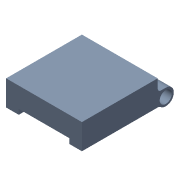
# Autodesk Inventor part: Rocker Box Top
Saved by Autodesk Inventor 2014 (Build 180170000, 170)
## iProperties
Created: 2013-05-18
Part Number: Rocker Box Top
Material: Generic
Document SubType Name: Modeling
Designer: richard
Density: 1 g/cm^3
Appearance: Light Steel Blue
Author: richard
Autodesk Inventor part; units mm, degrees
ref_plane "YZ Plane" through (0, 0, 0) normal (1, 0, 0) x (0, 1, 0)
ref_plane "XZ Plane" through (0, 0, 0) normal (0, 1, 0) x (-1, 0, 0)
ref_plane "XY Plane" through (0, 0, 0) normal (0, 0, 1) x (1, 0, 0)
sketch "Sketch1" plane through (0, 0, 0) normal (0, 0, 1) x (1, 0, 0)
  line L0 (-37.5, -5) -> (-25, -5)
  line L1 (-25, -5) -> (-25, 0)
  line L2 (-25, 0) -> (25, 0)
  line L3 (25, 0) -> (25, -5)
  line L4 (25, -5) -> (37.5, -5)
  line L5 (37.5, -5) -> (37.5, 20)
  line L6 (37.5, 20) -> (-37.5, 20)
  line L7 (-37.5, 20) -> (-37.5, -5)
  line L8 (0, 20) -> (0, 0) construction
  dimension "d0" = 50
  dimension "d1" = 75
  dimension "d2" = 25
  dimension "d3" = 5
  constraints: 18 end point, 5 parallel, 3 midpoint, 2 collinear, 2 perpendicular, 1 coincident, 1 horizontal, 1 other
  measures "d0" distance of L1.end L2.end
  measures "d1" distance between parallel lines of L5 L7
  measures "d2" distance between parallel lines of L6 L4
  measures "d3" distance of L2.end L3.end
extrude "Extrusion1" add sketch "Sketch1" along normal blind 75
sketch "Sketch2" plane through (-25, 0, 0) normal (0, -1, 0) x (1, 0, 0)
  line L0 (50, 0) -> (50, 75) projected
  line L1 (0, 0) -> (0, 75) projected
  line L2 (0, 37.5) -> (50, 37.5)
  line L3 (15, 37.5) -> (15, 48.6803)
  line L4 (35, 37.5) -> (35, 48.6803)
  line L5 (25, 37.5) -> (25, 52.5) construction
  arc A0 (35, 48.6803) -> (15, 48.6803) centre (25, 37.5) ccw
  point P0 (25, 0)
  dimension "d7" = 15
  dimension "d8" = 20
  constraints: 8 end point, 3 midpoint, 3 point on circle, 2 parallel, 2 point on line, 1 centre point, 1 perpendicular, 1 other
  measures "d7" radius of A0
  measures "d8" distance between parallel lines of L4 L3
revolve "Revolution1" cut sketch "Sketch2" angle 360 about axis through (-25, 0, 37.5) along (1, 0, 0)
sketch "Sketch4" plane through (37.5, -5, 0) normal (1, 0, 0) x (0, 0, -1)
  line L0 (0, 0) -> (0, 25) projected
  line L1 (0, 5) -> (0, 13)
  circle A0 centre (8, 5) radius 6
  arc A1 (1.755, 0) -> (8, 13) centre (8, 5) ccw
  line L2 (0, 13) -> (8, 13)
  line L3 (0, 0) -> (-75, 0) projected
  line L4 (0, 0) -> (1.755, 0)
  line L5 (0, 0) -> (0, 5)
  dimension "d18" = 12
  dimension "d19" = 2
  constraints: 8 end point, 2 centre point, 2 collinear, 2 point on circle, 2 tangent, 1 coincident, 1 perpendicular, 1 point on line
  measures "d18" diameter of A0
  measures "d19" radial gap between concentric circles of A1 A0
extrude "Extrusion3" add sketch "Sketch4" against normal up to surface (12.5 mm away) from surface at 0
fillet "Fillet2" radius 3 2 edges at (31.25, 8, 0) (31.25, -5, -1.755)
mirror "Mirror2" about plane through (0, 0, 0) normal (1, 0, 0) of "Extrusion3", "Fillet2"
body "Solid1"
